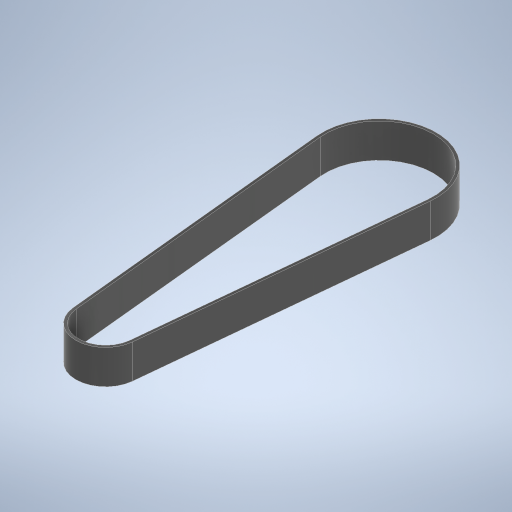
# Autodesk Inventor part: 2309HCMUTE-CDT23-BELT_S5M-355X71X15
Saved by Autodesk Inventor 2023 (Build 270158000, 158)
## iProperties
Created: 2023-11-01
Part Number: 2309HCMUTE-CDT23-BELT_S5M-355X71X15
Material: Rubber
Document SubType Name: Modeling
Designer: havie
Density: 0.93 g/cm^3
Appearance: Dark Gray
Author: havie
Autodesk Inventor part; units mm, degrees
ref_plane "YZ Plane" through (0, 0, 0) normal (1, 0, 0) x (0, 1, 0)
ref_plane "XZ Plane" through (0, 0, 0) normal (0, 1, 0) x (-1, 0, 0)
sketch "Sketch1" plane through (0, 0, 0) normal (0, 1, 0) x (-1, 0, 0)
  arc A0 (11.8839, 1.1821) -> (-11.8839, 1.1821) centre (0, 0) ccw
  arc A1 (-23.7682, -118.2958) -> (23.7682, -118.2958) centre (0, -120.66) ccw
  line L0 (11.8839, 1.1821) -> (23.7682, -118.2958)
  line L1 (-11.8839, 1.1821) -> (-23.7682, -118.2958)
  dimension "d0" = 23.885
  dimension "d1" = 47.771
  dimension "d2" = 120.66
  constraints: 4 end point, 4 point on circle, 4 tangent, 2 centre point, 1 coincident, 1 vertical alignment
  measures "d0" diameter of A0
  measures "d1" diameter of A1
  measures "d2" distance of point (0, 0) A1.centre
ref_plane "Work Plane1" through (-11.8839, 0, 1.1821) normal (-0.0989806, 0, -0.9950894) x (0, -1, 0)
sketch "Sketch2" plane through (-11.8839, 0, 1.1821) normal (-0.0989806, 0, -0.9950894) x (0, -1, 0)
  line L0 (-7.5, 1.2) -> (7.5, 1.2)
  line L1 (7.5, 1.2) -> (7.5, 0)
  line L2 (7.5, 0) -> (-7.5, 0)
  line L3 (-7.5, 0) -> (-7.5, 1.2)
  line L4 (-7.5, 1.2) -> (7.5, 0) construction
  line L5 (7.5, 1.2) -> (-7.5, 0) construction
  point P0 (0, -11.9425)
  point P1 (0, 0.6)
  point P2 (0, 0)
  point P3 (0, 0)
  dimension "d3" = 1.2
  dimension "d4" = 15
  constraints: 12 end point, 3 midpoint, 2 parallel, 1 coincident, 1 horizontal, 1 perpendicular
  measures "d3" distance of L2.end L0.start
  measures "d4" distance of L0.start L0.end
sweep "Sweep1" add profiles "Sketch2" path "Sketch1"
body "Solid1"
